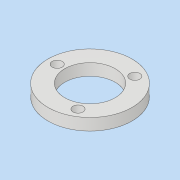
# Autodesk Inventor part: SmallSpoolExpander
Saved by Autodesk Inventor 2017.3 (Build 213256000, 256)
## iProperties
Created: 2019-01-16
Part Number: SmallSpoolExpander
Material: ABS Plastic
Document SubType Name: Modeling
Designer: Derek Wider
Density: 1.06 g/cm^3
Appearance: Smooth - White
Author: Derek Wider
Autodesk Inventor part; units mm, degrees
ref_plane "YZ Plane" through (0, 0, 0) normal (1, 0, 0) x (0, 1, 0)
ref_plane "XZ Plane" through (0, 0, 0) normal (0, 1, 0) x (-1, 0, 0)
ref_plane "XY Plane" through (0, 0, 0) normal (0, 0, 1) x (1, 0, 0)
sketch "Sketch1" plane through (0, 0, 0) normal (0, 1, 0) x (-1, 0, 0)
  circle A0 centre (0, 0) radius 15.875
  line L0 (0, 0) -> (12.3952, 0)
  circle A1 centre (12.3952, 0) radius 1.905
  circle A2 centre (0, 0) radius 9.525
  circle A3 centre (-6.1976, 10.7346) radius 1.905
  circle A4 centre (-6.1976, -10.7346) radius 1.905
  dimension "d0" = 31.75
  dimension "d1" = 12.3952
  dimension "d2" = 3.81
  dimension "d3" = 19.05
  dimension "d6" = 360
  constraints: 5 centre point, 3 coincident, 2 end point, 1 horizontal, 7 other
  measures "d0" diameter of A0
  measures "d1" distance of L0.start L0.end
  measures "d2" diameter of A1
  measures "d3" diameter of A2
extrude "Extrusion1" add sketch "Sketch1" along normal blind 4.445
body "Solid1"
